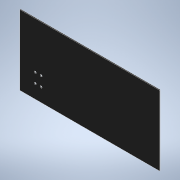
# Autodesk Inventor part: 後ろカバー
Saved by Autodesk Inventor 2022 (Build 260153000, 153)
## iProperties
Created: 2022-11-07
Part Number: 後ろカバー
Material: ABS プラスチック
Document SubType Name: Modeling
Designer: tdn82
Density: 1.06 g/cm^3
Appearance: 滑らか - 白
Author: tdn82
Autodesk Inventor part; units mm, degrees
ref_plane "YZ Plane" through (0, 0, 0) normal (1, 0, 0) x (0, 1, 0)
ref_plane "XZ Plane" through (0, 0, 0) normal (0, 1, 0) x (-1, 0, 0)
ref_plane "XY Plane" through (0, 0, 0) normal (0, 0, 1) x (1, 0, 0)
sketch "スケッチ1" plane through (0, 0, 0) normal (0, 0, 1) x (1, 0, 0)
  line L0 (0, 0) -> (360, 0)
  line L1 (360, 0) -> (360, -180)
  line L2 (360, -180) -> (0, -180)
  line L3 (0, -180) -> (0, 0)
  dimension "d0" = 360
  dimension "d1" = 180
  constraints: 8 end point, 2 parallel, 1 horizontal, 1 perpendicular
  measures "d0" distance of L0.start L0.end
  measures "d1" distance of L2.end L0.start
extrude "押し出し1" add sketch "スケッチ1" along normal blind 2
sketch "スケッチ3" plane through (0, 0, 2) normal (0, 0, 1) x (1, 0, 0)
  line L0 (360, 0) -> (0, 0) projected
  line L1 (0, 0) -> (0, -180) projected
  point P0 (55, -145)
  point P1 (30, -145)
  point P2 (55, -120)
  point P3 (30, -120)
  dimension "d14" = 145
  dimension "d15" = 55
  dimension "d18" = 25
  dimension "d21" = 25
  constraints: 1 horizontal, 1 vertical, 3 other
  measures "d14" distance from line of L0 point (55, -145)
  measures "d15" distance from line of L1 point (55, -145)
  measures "d18" distance of point (55, -145) point (30, -145)
  measures "d21" distance of point (55, -145) point (55, -120)
hole "穴2" at (55, -145, 2) at (30, -145, 2) at (55, -120, 2) at (30, -120, 2) direction (0, 0, -1) diameter 3.5 end through all
